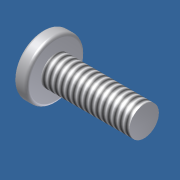
# Autodesk Inventor part: HW-00015
Saved by Autodesk Inventor 2012 (Build 160160000, 160)
## iProperties
Created: 2008-09-25
Part Number: HW-00015
Document SubType Name: Modeling
Designer: mcyr
Density: 1 g/cm^3
Description: 1/4-20 x 3/4" Button head screw, zinc plated
Mass: 0.985611 g
Surface Area: 8.13131 cm^2
Volume: 0.985611 cm^3
Material: Default
Author: mcyr
Autodesk Inventor part; units mm, degrees
ref_plane "YZ Plane" through (0, 0, 0) normal (1, 0, 0) x (0, 1, 0)
ref_plane "XZ Plane" through (0, 0, 0) normal (0, 1, 0) x (-1, 0, 0)
ref_plane "XY Plane" through (0, 0, 0) normal (0, 0, 1) x (1, 0, 0)
sketch "Sketch1" plane through (0, 0, 0) normal (0, 0, 1) x (1, 0, 0)
  line L0 (-10.5828, 0.0599) -> (12.7085, 0.0599)
  line L1 (12.7085, 0.0599) -> (12.7085, 3.2349)
  line L2 (12.7085, 3.2349) -> (-6.3415, 3.2349)
  line L3 (-6.3415, 3.2349) -> (-6.3415, 5.715)
  line L4 (-6.9765, 6.35) -> (-8.5085, 6.35)
  arc A0 (-9.0678, 6.0158) -> (-10.5828, 0.0599) centre (2.1171, 0) ccw
  arc A1 (-6.3415, 5.715) -> (-6.9765, 6.35) centre (-6.9765, 5.715) ccw
  arc A2 (-8.5085, 6.35) -> (-9.0678, 6.0158) centre (-8.5085, 5.715) ccw
  point P0 (-6.3415, 6.35)
  dimension "d1" = 3.175
  dimension "d3" = 19.05
  dimension "d6" = 12.7
  dimension "d8" = 0.635
  constraints: 10 end point, 6 point on circle, 4 tangent, 3 centre point, 3 parallel, 2 point on line, 1 equal radius, 1 horizontal, 1 perpendicular
  measures "d1" distance of L0.end L1.end
  measures "d3" distance of L1.end L2.end
  measures "d6" radius of A0
  measures "d8" radius of A1
revolve "Revolution1" add sketch "Sketch1" angle 360 about axis through (-10.5828, 0.0599, 0) along (1, 0, 0)
thread "Thread1" size "1/4-20 UNC" class "2A" standard "ANSI Unified Screw Threads" full length
sketch "Sketch2" plane through (-6.3415, 0.0599, 0) normal (1, 0, 0) x (0, 0, -1)
  line L0 (0.4205, -2.6234) -> (-0.4685, -2.6234)
  line L1 (-0.4685, -2.6234) -> (-0.4685, 2.8376)
  line L2 (-0.4685, 2.8376) -> (0.4205, 2.8376)
  line L3 (0.4205, 2.8376) -> (0.4205, -2.6234)
  line L4 (2.7065, -0.3374) -> (-2.7545, -0.3374)
  line L5 (-2.7545, -0.3374) -> (-2.7545, 0.5516)
  line L6 (-2.7545, 0.5516) -> (2.7065, 0.5516)
  line L7 (2.7065, 0.5516) -> (2.7065, -0.3374)
  dimension "d12" = 0.889
  dimension "d13" = 0.889
  dimension "d20" = 2.286
  dimension "d21" = 2.286
  dimension "d22" = 2.286
  dimension "d23" = 2.286
  constraints: 16 end point, 4 parallel, 2 horizontal, 2 perpendicular
  measures "d12" distance of L6.end L4.start
  measures "d13" distance of L0.start L0.end
  measures "d20" horizontal distance of L0.end L4.end
  measures "d21" horizontal distance of L0.start L4.start
  measures "d22" horizontal distance of L4.start L0.start
  measures "d23" horizontal distance of L5.end L1.end
extrude "Extrusion1" cut sketch "Sketch2" against normal blind 4.445
body "Solid1"
